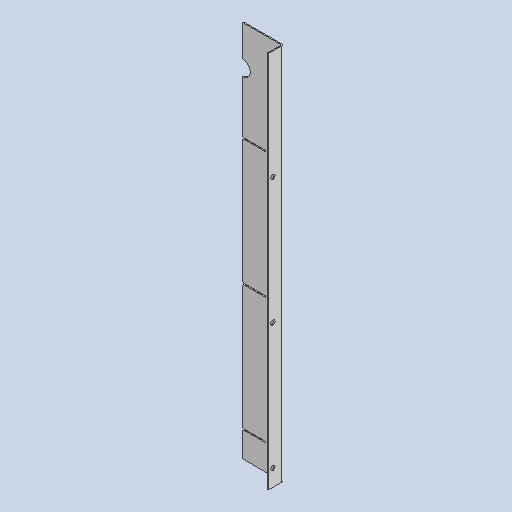
# Autodesk Inventor part: GBK 0202 stringer 4
Saved by Autodesk Inventor 2026.2 (Build 302298000, 298)
## iProperties
Created: 2026-05-07
Part Number: GBK 0202 stringer 4
Material: Steel
Document SubType Name: Sheet Metal
Designer: pokla
Density: 7.85 g/cm^3
Sheet Metal Rule: Default_mm
Appearance: Default
Mass: 9714.66 g
Surface Area: 6353.15 cm^2
Volume: 1237.54 cm^3
Flat Pattern Width: 20.9726 cm
Flat Pattern Length: 148.95 cm
Flat Pattern Area: 3123.87 cm^2
Sheet Metal Width: 209,726 mm
Sheet Metal Length: 1489,500 mm
Sheet Metal Area: 312386,862 mm^2
Stock Number: 0202
Description: 3
Author: admin
Autodesk Inventor part; units mm, degrees
ref_plane "YZ Plane" through (0, 0, 0) normal (1, 0, 0) x (0, 1, 0)
ref_plane "XZ Plane" through (0, 0, 0) normal (0, 1, 0) x (-1, 0, 0)
ref_plane "XY Plane" through (0, 0, 0) normal (0, 0, 1) x (1, 0, 0)
sketch "Sketch1" plane through (0, 0, 0) normal (0, 0, 1) x (1, 0, 0)
  line L0 (0, 0) -> (-156.6782, 0)
  line L1 (-156.6782, 0) -> (-156.6782, -1489.5)
  line L2 (-156.6782, -1489.5) -> (0, -1489.5)
  line L3 (0, -1489.5) -> (0, 0)
  line L4 (-156.6782, -1389.5) -> (-66, -1389.5)
  line L5 (-66, -1389.5) -> (-66, -1384.5)
  line L6 (-66, -1384.5) -> (-156.6782, -1384.5)
  line L7 (-156.6782, -1384.5) -> (-156.6782, -1389.5)
  line L8 (-156.6782, -892.8333) -> (-66, -892.8333)
  line L9 (-66, -892.8333) -> (-66, -887.8333)
  line L10 (-66, -887.8333) -> (-156.6782, -887.8333)
  line L11 (-156.6782, -887.8333) -> (-156.6782, -892.8333)
  line L12 (-156.6782, -396.1667) -> (-66, -396.1667)
  line L13 (-66, -396.1667) -> (-66, -391.1667)
  line L14 (-66, -391.1667) -> (-156.6782, -391.1667)
  line L15 (-156.6782, -391.1667) -> (-156.6782, -396.1667)
  circle A0 centre (-156.6782, -154.5) radius 30
  point P0 (-156.6782, -1384.5)
  point P1 (-156.6782, -124.5)
  point P2 (-156.6782, -184.5)
  dimension "d0" = 1489.5
  dimension "d1" = 156.6782
  dimension "d2" = 5
  dimension "d4" = 100
  dimension "d7" = 496.6667
  dimension "d23" = 66
  dimension "d28" = 60
  dimension "d29" = 1335
  measures "d0" distance of L1.end L0.end
  measures "d1" distance of L1.end L2.end
  measures "d2" distance of L4.end L5.end
  measures "d4" distance between parallel lines of L2 L4
  measures "d7" distance of L4.start L8.start
  measures "d23" distance between parallel lines of L3 L5
  measures "d28" diameter of A0
  measures "d29" distance from line of L2 A0.centre
extrude "Plate1" add sketch "Sketch1" along normal blind 4 contours L3 L2 L1 L4 L5 L6 L8 L9 L10 L12 L13 L14 A0 L0
sketch "Sketch2" plane through (-4, 0, 0) normal (1, 0, 0) x (0, 1, 0)
  line L0 (-1489.5, 0) -> (0, 0)
  line L1 (0, 0) -> (0, 60)
  line L2 (0, 60) -> (-1489.5, 60)
  line L3 (-1489.5, 60) -> (-1489.5, 0)
  constraints: 6 end point, 1 horizontal, 1 perpendicular, 1 vertical
edge flange "Flange1" height 60 angle 90 thickness 4 bend radius 4 thickness toward (1, 0, 0) relief straight relief width 4 relief depth 2 edges at (0, -744.75, 4) wall of the first edge with corners at (-4, -1489.5, 0) (-4, 0, 0) (-4, 0, 60) (-4, -1489.5, 60)
bend "Bend1"
corner "Corner1"
chamfer "Corner Chamfer1" distance 3 angle 45 6 edges at (-156.6782, -1389.5, 2) (-156.6782, -1384.5, 2) (-156.6782, -892.8333, 2) (-156.6782, -887.8333, 2) (-156.6782, -391.1667, 2) (-156.6782, -396.1667, 2)
sketch "Sketch4" plane through (0, -1489.5, 60) normal (1, 0, 0) x (0, 0, -1)
  circle A0 centre (18, 1059.5) radius 9
  line L0 (0, 0) -> (0, 1489.5) projected
  circle A1 centre (18, 562.8333) radius 9
  circle A2 centre (18, 66.1667) radius 9
  point P0 (60, 1489.5)
  dimension "d30" = 18
  dimension "d31" = 18
  dimension "d32" = 430
  dimension "d35" = 496.6667
  constraints: 3 centre point, 1 vertical, 4 other
  measures "d30" distance from line of A0.centre L0
  measures "d31" diameter of A0
  measures "d32" vertical distance of point (60, 1489.5) A0.centre
  measures "d35" distance of A0.centre A1.centre
extrude "Cut1" cut sketch "Sketch4" against normal blind 4
equation "\"d0\" = Стрингер_длина"
equation "\"d1\" = стрингер_глубина_4"
equation "\"d2\" = паз_под_стрингер_толщина"
equation "\"d7\" = Шаг_шпангоутов"
equation "\"d23\" = паз_под_стрингер_глубина - Thickness"
equation "\"d28\" = 2 * радиус_выреза_под_сварку"
equation "\"d35\" = Шаг_шпангоутов"
equation "\"d40\" = Thickness"
equation "\"d12\" = Thickness"
equation "\"d13\" = BendReliefWidth"
equation "\"d14\" = BendReliefDepth"
equation "\"d15\" = MinimumRemnant"
equation "\"d16\" = TransitionRadius"
equation "\"d17\" = ребро_усилителей"
equation "\"d19\" = BendRadius"
equation "\"d20\" = CornerReliefSize"
equation "\"d21\" = GapSize"
equation "\"d22\" = JacobiRadiusSize"
equation "\"BendRadius\" = Thickness"
equation "\"BendReliefWidth\" = Thickness"
equation "\"BendReliefDepth\" = 0.5 * Thickness"
equation "\"CornerReliefSize\" = 4 * Thickness"
equation "\"MinimumRemnant\" = 2 * Thickness"
equation "\"TransitionRadius\" = BendRadius"
equation "\"JacobiRadiusSize\" = BendRadius"
equation "\"GapSize\" = Thickness"
equation "\"Стрингер_длина\" = 1489.5"
equation "\"стрингер_глубина_4\" = 156.678203"
equation "\"паз_под_стрингер_толщина\" = 5"
equation "\"Шаг_шпангоутов\" = 496.666667"
equation "\"паз_под_стрингер_глубина\" = 70"
equation "\"Thickness\" = 4"
equation "\"радиус_выреза_под_сварку\" = 30"
equation "\"ребро_усилителей\" = 60"
body "Solid1"
